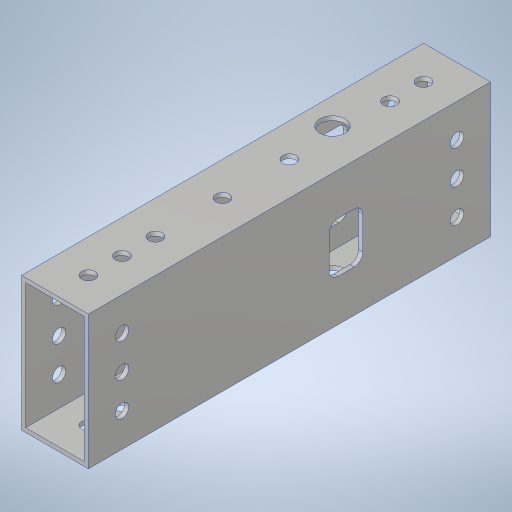
# Autodesk Inventor part: EL2-C-005
Saved by Autodesk Inventor 2023.4 (Build 274418000, 418)
## iProperties
RuleStatus: InUse
Created: 2025-01-11
Part Number: EL2-C-005
Material: Aluminum 6061
Document SubType Name: Modeling
Designer: brand
Mass: 304.185 g
Surface Area: 718.547 cm^2
Volume: 112.661 cm^3
Density: 2.7 g/cm^3
Appearance: Aluminum - Flat
AfterDocNew0: SHOW
AfterDocOpen0: SHOW
Author: brand
Autodesk Inventor part; units mm, degrees
ref_plane "YZ Plane" through (0, 0, 0) normal (1, 0, 0) x (0, 1, 0)
ref_plane "XZ Plane" through (0, 0, 0) normal (0, 1, 0) x (-1, 0, 0)
ref_plane "XY Plane" through (0, 0, 0) normal (0, 0, 1) x (1, 0, 0)
sketch "Sketch1" plane through (0, 0, 0) normal (0, 0, 1) x (1, 0, 0)
  line L0 (-12.7, -25.4) -> (12.7, -25.4)
  line L1 (12.7, -25.4) -> (12.7, 25.4)
  line L2 (12.7, 25.4) -> (-12.7, 25.4)
  line L3 (-12.7, 25.4) -> (-12.7, -25.4)
  line L4 (-12.7, -25.4) -> (12.7, 25.4) construction
  line L5 (12.7, -25.4) -> (-12.7, 25.4) construction
  line L6 (-11.1125, 23.8125) -> (11.1125, 23.8125)
  line L7 (11.1125, 23.8125) -> (11.1125, -23.8125)
  line L8 (11.1125, -23.8125) -> (-11.1125, -23.8125)
  line L9 (-11.1125, -23.8125) -> (-11.1125, 23.8125)
  point P0 (0, 0)
  dimension "width" = 25.4
  dimension "height" = 50.8
  dimension "thickness" = 1.5875
  constraints: 20 end point, 4 parallel, 2 midpoint, 2 perpendicular, 1 horizontal, 3 other
  measures "width" distance of L2.end L1.end
  measures "height" distance of L1.end L0.end
  measures "thickness" distance between parallel lines of L2 L6
extrude "Extrusion1" add sketch "Sketch1" along normal mid plane 152.4
sketch "Sketch2" plane through (-12.7, -25.4, 76.2) normal (-1, 0, 0) x (0, 0, 1)
  line L0 (-152.4, 0) -> (-152.4, 50.8) construction
  line L1 (-152.4, 50.8) -> (0, 50.8) construction
  line L2 (0, 50.8) -> (0, 0) construction
  line L3 (0, 0) -> (-152.4, 0) construction
  point P0 (-76.2, 25.4)
  point P1 (-139.7, 38.1)
  point P2 (-139.7, 25.4)
  point P3 (-139.7, 12.7)
  point P4 (-12.7, 38.1)
  point P5 (-12.7, 25.4)
  point P6 (-12.7, 12.7)
  point P7 (-152.4, 25.4)
  dimension "d5" = 12.7
  dimension "d6" = 12.7
  dimension "d7" = 12.7
  dimension "d8" = 12.7
  constraints: 4 horizontal alignment, 4 vertical alignment, 1 midpoint
  measures "d5" distance of point (-139.7, 38.1) point (-139.7, 25.4)
  measures "d6" distance of point (-139.7, 12.7) point (-139.7, 25.4)
  measures "d7" distance from line of L0 point (-139.7, 25.4)
  measures "d8" distance from line of L2 point (-12.7, 25.4)
hole "Hole1" at (-12.7, 12.7, -63.5) at (-12.7, 0, -63.5) at (-12.7, -12.7, -63.5) at (-12.7, 12.7, 63.5) at (-12.7, 0, 63.5) at (-12.7, -12.7, 63.5) direction (1, 0, 0) diameter 5.1054 end through all clearance for "Flat Head Machine Screw (82)" size "#10" standard "Ansi Unified Screw Threads"
sketch "Sketch3" plane through (-12.7, 25.4, 76.2) normal (0, 1, 0) x (1, 0, 0)
  line L0 (0, 152.4) -> (25.4, 152.4) construction
  line L1 (25.4, 152.4) -> (25.4, 0) construction
  line L2 (25.4, 0) -> (0, 0) construction
  line L3 (0, 0) -> (0, 152.4) construction
  line L4 (25.4, 152.4) -> (25.4, 0) construction
  line L5 (25.4, 0) -> (0, 0) construction
  line L6 (0, 0) -> (0, 152.4) construction
  line L7 (0, 152.4) -> (25.4, 152.4) projected
  point P0 (12.7, 76.2)
  point P1 (12.7, 12.7)
  point P2 (12.7, 0)
  dimension "d16" = 12.7
  constraints: 1 midpoint, 1 vertical alignment
  measures "d16" distance from line of L2 point (12.7, 12.7)
hole "Hole2" at (0, 25.4, 63.5) direction (0, -1, 0) diameter 5.1054 end through all clearance for "Flat Head Machine Screw (82)" size "#10" standard "Ansi Unified Screw Threads"
pattern_linear "Rectangular Pattern1" count 4 spacing 25.4 along (0, 0, -1) of "Hole2"
sketch "Sketch4" plane through (-12.7, 25.4, 76.2) normal (0, 1, 0) x (1, 0, 0)
  circle A0 centre (12.7, 12.7) radius 2.5527 projected
  line L0 (0, 152.4) -> (25.4, 152.4) projected
  point P0 (12.7, 76.2)
  point P1 (12.7, 25.4)
  point P2 (12.7, 127)
  point P3 (12.7, 152.4)
  point P4 (12.7, 139.7)
  dimension "d27" = 12.7
  dimension "d44" = 25.4
  dimension "d52" = 12.7
  constraints: 3 vertical alignment, 1 midpoint
  measures "d27" distance of A0.centre point (12.7, 25.4)
  measures "d44" distance of point (12.7, 152.4) point (12.7, 127)
  measures "d52" distance from line of L0 point (12.7, 139.7)
hole "Hole3" at (0, 25.4, 50.8) at (0, 25.4, -50.8) at (0, 25.4, -63.5) direction (0, -1, 0) diameter 5.1054 end through all clearance for "Flat Head Machine Screw (82)" size "#10" standard "Ansi Unified Screw Threads"
sketch "Sketch5" plane through (-12.7, -25.4, 76.2) normal (-1, 0, 0) x (0, 0, 1)
  line L0 (-121.92, 9.525) -> (-93.98, 9.525)
  line L1 (-93.98, 9.525) -> (-93.98, 41.275)
  line L2 (-93.98, 41.275) -> (-121.92, 41.275)
  line L3 (-121.92, 41.275) -> (-121.92, 9.525)
  line L4 (-152.4, 0) -> (-152.4, 50.8) projected
  point P0 (-76.2, 25.4)
  point P1 (-121.92, 25.4)
  point P2 (-152.4, 25.4)
  point P3 (-107.95, 9.525)
  dimension "d36" = 30.48
  dimension "d37" = 31.75
  dimension "d38" = 27.94
  constraints: 8 end point, 3 midpoint, 2 parallel, 1 horizontal, 1 horizontal alignment, 1 perpendicular
  measures "d36" distance between parallel lines of L4 L3
  measures "d37" distance from line of L2 point (-107.95, 9.525)
  measures "d38" distance between parallel lines of L3 L1
extrude "Extrusion2" cut sketch "Sketch5" against normal blind 1.5875
fillet "Fillet1" radius 3.302 4 edges at (-11.9062, -15.875, -45.72) (-11.9062, 15.875, -45.72) (-11.9062, 15.875, -17.78) (-11.9062, -15.875, -17.78)
sketch "Sketch6" plane through (-12.7, -25.4, 76.2) normal (0, -1, 0) x (1, 0, 0)
  line L0 (25.4, -152.4) -> (0, -152.4) projected
  line L1 (0, 0) -> (0, -152.4) projected
  point P0 (12.7, -76.2)
  point P1 (9.9314, -107.95)
  point P2 (12.7, -152.4)
  dimension "d43" = 44.45
  dimension "d53" = 9.9314
  constraints: 1 midpoint
  measures "d43" distance from line of L0 point (9.931, -107.95)
  measures "d53" distance from line of L1 point (9.931, -107.95)
hole "Hole4" at (-2.7686, -25.4, -31.75) direction (0, 1, 0) diameter 9.525 end through all
sketch "Sketch7" plane through (12.7, -25.4, 76.2) normal (1, 0, 0) x (0, 0, -1)
  line L0 (152.4, 50.8) -> (152.4, 0) projected
  line L1 (103.9876, 34.925) -> (91.2876, 34.925)
  line L2 (91.2876, 34.925) -> (91.2876, 15.875)
  line L3 (91.2876, 15.875) -> (103.9876, 15.875)
  line L4 (103.9876, 15.875) -> (103.9876, 34.925)
  line L5 (103.9876, 34.925) -> (91.2876, 15.875) construction
  line L6 (91.2876, 34.925) -> (103.9876, 15.875) construction
  point P0 (76.2, 25.4)
  point P1 (97.6376, 25.4)
  point P2 (152.4, 25.4)
  dimension "d55" = 54.7624
  dimension "d56" = 12.7
  dimension "d57" = 19.05
  constraints: 12 end point, 3 midpoint, 2 parallel, 1 horizontal, 1 horizontal alignment, 1 perpendicular
  measures "d55" distance from line of L0 point (97.638, 25.4)
  measures "d56" distance of L1.start L1.end
  measures "d57" distance of L1.end L2.end
extrude "Extrusion3" cut sketch "Sketch7" against normal blind 1.5875
fillet "Fillet2" radius 3.302 4 edges at (11.9062, 9.525, -27.7876) (11.9062, -9.525, -27.7876) (11.9062, -9.525, -15.0876) (11.9062, 9.525, -15.0876)
equation "\"d6\" = d5"
equation "\"d8\" = d7"
body "Solid1"
